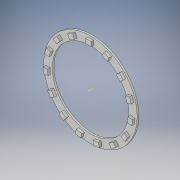
# Autodesk Inventor part: Light Ring
Saved by Autodesk Inventor 2019 (Build 230136000, 136)
## iProperties
Created: 2019-01-11
Part Number: Light Ring
Material: Generic
Document SubType Name: Modeling
Designer: pepin
Density: 1 g/cm^3
Appearance: Default
Author: pepin
Autodesk Inventor part; units mm, degrees
ref_plane "YZ Plane" through (0, 0, 0) normal (1, 0, 0) x (0, 1, 0)
ref_plane "XZ Plane" through (0, 0, 0) normal (0, 1, 0) x (-1, 0, 0)
ref_plane "XY Plane" through (0, 0, 0) normal (0, 0, 1) x (1, 0, 0)
sketch "Sketch1" plane through (0, 0, 0) normal (0, 0, 1) x (1, 0, 0)
  circle A0 centre (0, 0) radius 24.5
  circle A1 centre (0, 0) radius 30
  dimension "d0" = 49
  dimension "d1" = 60
  constraints: 2 centre point, 2 coincident
  measures "d0" diameter of A0
  measures "d1" diameter of A1
extrude "Extrusion1" add sketch "Sketch1" against normal blind 1.1
sketch "Sketch2" plane through (0, 0, 0) normal (0, 0, 1) x (1, 0, 0)
  line L0 (0, 0) -> (0, 30) construction
  circle A0 centre (0, 0) radius 30 construction
  line L1 (-1.73, 27.25) -> (2.3469, 27.25) construction
  line L2 (2.3469, 27.25) -> (2.3469, 25.3632) construction
  line L3 (2.3469, 25.3632) -> (-1.73, 25.3632) construction
  line L4 (-1.73, 25.3632) -> (-1.73, 27.25) construction
  line L5 (-1.4916, 25.85) -> (2.1084, 25.85)
  line L6 (2.1084, 25.85) -> (2.1084, 28.65)
  line L7 (2.1084, 28.65) -> (-1.4916, 28.65)
  line L8 (-1.4916, 28.65) -> (-1.4916, 25.85)
  line L9 (-1.4916, 25.85) -> (2.1084, 28.65) construction
  line L10 (2.1084, 25.85) -> (-1.4916, 28.65) construction
  point P0 (0.3084, 27.25)
  dimension "d4" = 27.25
  dimension "d5" = 2.8
  dimension "d6" = 3.6
  constraints: 22 end point, 5 parallel, 3 midpoint, 2 perpendicular, 1 horizontal, 1 vertical, 1 vertical alignment, 1 other
  measures "d4" vertical distance of point (0.308, 27.25) L0.start
  measures "d5" distance of L5.end L6.end
  measures "d6" distance of L5.start L5.end
extrude "Extrusion2" add sketch "Sketch2" along normal blind 1.7
pattern_circular "Circular Pattern1" count 15 over 360 about axis through (0, 0, -10) along (0, 0, 1) of "Extrusion2"
body "Solid1"
